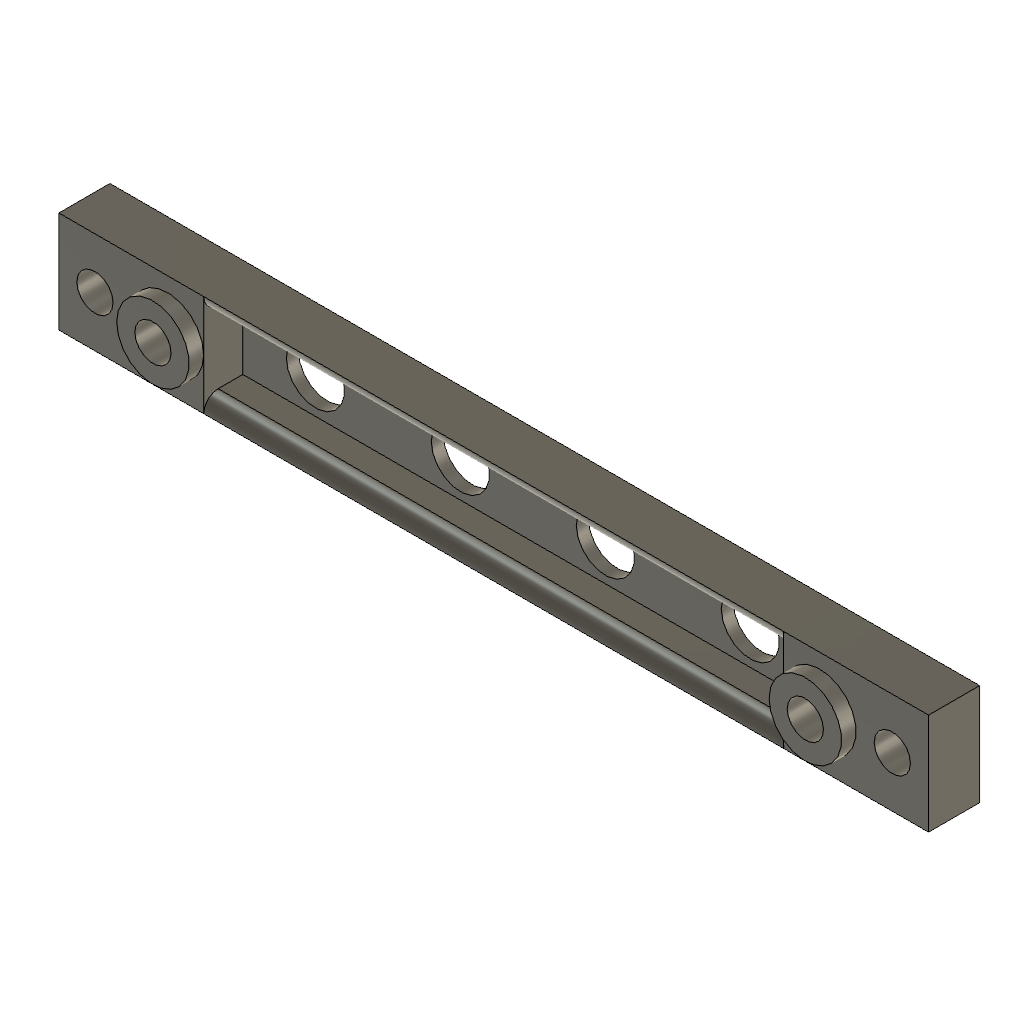
Button Plate (Autodesk Fusion 360 design; units mm, degrees)
Autodesk Fusion 360 part; units mm, degrees
note: some values were not read from the file. Set by a fixed rule: which sketch regions a step uses.
sketch "Sketch1" plane through (0, 0, 0) normal (0, 1, 0) x (1, 0, 0)
  line L0 (0, 0) -> (60, 0)
  line L1 (60, 0) -> (60, -7)
  line L2 (60, -7) -> (0, -7)
  line L3 (0, -7) -> (0, 0)
  line L4 (0, -7) -> (2.5, -7)
  line L5 (2.5, -7) -> (2.5, -3.5)
  line L6 (2.5, -3.5) -> (0, -3.5)
  line L7 (0, -3.5) -> (0, -7)
  line L8 (60, -7) -> (57.5, -7)
  line L9 (57.5, -7) -> (57.5, -3.5)
  line L10 (57.5, -3.5) -> (60, -3.5)
  line L11 (60, -3.5) -> (60, -7)
  circle A0 centre (2.5, -3.5) radius 1.25
  circle A1 centre (57.5, -3.5) radius 1.25
  line L12 (0, -7) -> (30, -7)
  line L13 (0, -7) -> (18, -7)
  line L14 (60, -7) -> (42, -7)
  line L15 (2.5, -3.5) -> (7.5, -3.5)
  line L16 (57.5, -3.5) -> (52.5, -3.5)
  circle A2 centre (7.5, -3.5) radius 1.25
  circle A3 centre (52.5, -3.5) radius 1.25
  circle A4 centre (52.5, -3.5) radius 2.5
  circle A5 centre (7.5, -3.5) radius 2.5
  line L17 (7.5, -3.5) -> (15, -3.5)
  line L18 (52.5, -3.5) -> (45, -3.5)
  line L19 (15, -3.5) -> (25, -3.5)
  line L20 (25, -3.5) -> (35, -3.5)
  line L21 (35, -3.5) -> (45, -3.5)
  circle A6 centre (15, -3.5) radius 2
  circle A7 centre (25, -3.5) radius 2
  circle A8 centre (35, -3.5) radius 2
  circle A9 centre (45, -3.5) radius 2
  dimension "d1" = 60
  dimension "d2" = 7
  dimension "d3" = 2.5
  dimension "d4" = 3.5
  dimension "d5" = 2.5
  dimension "d6" = 3.5
  dimension "d7" = 2.5
  dimension "d8" = 2.5
  dimension "d79" = 5
  dimension "d80" = 5
  dimension "d81" = 2.5
  dimension "d82" = 2.5
  dimension "d83" = 5
  dimension "d84" = 5
  dimension "d85" = 7.5
  dimension "d86" = 7.5
  dimension "d87" = 10
  dimension "d88" = 10
  dimension "d89" = 10
  dimension "d90" = 4
  dimension "d91" = 4
  dimension "d92" = 4
  dimension "d93" = 4
  constraint horizontal L0
  constraint vertical L1
  constraint horizontal L2
  constraint vertical L3
  constraint coincident L0.start L3.end
  constraint horizontal L4
  constraint vertical L5
  constraint horizontal L6
  constraint vertical L7
  constraint horizontal L8
  constraint vertical L9
  constraint horizontal L10
  constraint vertical L11
  constraint coincident L5.end L6.start
  constraint coincident L9.end L10.start
  constraint perpendicular L7 L12
  constraint perpendicular L5 L13
  constraint perpendicular L11 L14
  constraint perpendicular L5 L15
  constraint perpendicular L9 L16
  constraint coincident L15.end A2.centre
  constraint coincident L16.end A3.centre
  constraint concentric A3 A4
  constraint concentric A2 A5
  constraint parallel L15 L17
  constraint parallel L16 L18
  constraint parallel L17 L19
  constraint parallel L19 L20
  constraint parallel L20 L21
  constraint coincident L17.end L19.start
  constraint coincident L19.end L20.start
  constraint coincident L20.end L21.start
  constraint coincident L18.end L21.end
  measures "d1" distance of L0.start L0.end
  measures "d2" distance of L0.start L2.end
  measures "d3" distance of L2.end L4.end
  measures "d4" distance of L2.end L6.end
  measures "d5" distance of L1.end L8.end
  measures "d6" distance of L1.end L10.end
  measures "d7" diameter of A0
  measures "d8" diameter of A1
  measures "d79" distance of L5.end L15.end
  measures "d80" distance of L9.end L16.end
  measures "d81" diameter of A2
  measures "d82" diameter of A3
  measures "d83" diameter of A4
  measures "d84" diameter of A5
  measures "d85" distance of L15.end L17.end
  measures "d86" distance of L16.end L18.end
  measures "d87" distance of L17.end L19.end
  measures "d88" distance of L19.end L20.end
  measures "d89" distance of L20.end L18.end
  measures "d90" diameter of A6
  measures "d91" diameter of A7
  measures "d92" diameter of A8
  measures "d93" diameter of A9
extrude "Extrude1" add sketch "Sketch1" along normal blind 3.532 contours L0 L1 L3 L6 L10 A0 A1 L15 L16 A4 A5 L17 L18 L19 L20 L21 A6 A7 A8 A9 | L2 L3 L4 L5 L6 L7 A0 L12 L13 | L1 L2 L8 L9 L10 L11 A1 L14 | L6 A0 L15 | L5 L6 A0 | L9 L10 A1 | L10 A1 L16 | L2 L5 L9 A0 A1 L12 L13 L14 L15 L16 A4 A5 L17 L18 L19 L20 L21 A6 A7 A8 A9 | L5 A0 L15 | L9 A1 L16 | L15 A2 A5 L17 | L15 A2 A5 L17 | L16 A3 A4 L18 | L16 A3 A4 L18 | L15 A2 L17 | L15 A2 L17 | L16 A3 L18 | L16 A3 L18
extrude "Extrude3" cut sketch "Sketch1" along normal blind 2 contours L6 A0 L15 | L5 L6 A0 | L9 L10 A1 | L10 A1 L16 | L5 A0 L15 | L9 A1 L16
extrude "Extrude4" add sketch "Sketch1" against normal blind 1 contours L15 A2 A5 L17 | L15 A2 A5 L17 | L16 A3 A4 L18 | L16 A3 A4 L18
extrude "Extrude12" cut 2 faces at (52.6522, 0, 3.8879) (7.2402, 0, 3.8258) along direction (0, 1, 0) blind 2
sketch "Sketch5" plane through (0, 0, 0) normal (0, -1, 0) x (1, 0, 0)
  circle A0 centre (7.5, 3.5) radius 2.5
  circle A1 centre (2.5, 3.5) radius 1.25
  circle A2 centre (57.5, 3.5) radius 1.25
  circle A3 centre (15, 3.5) radius 2
  circle A4 centre (45, 3.5) radius 2
  circle A5 centre (25, 3.5) radius 2
  circle A6 centre (35, 3.5) radius 2
  line L0 (0, 7) -> (0, 0)
  line L1 (0, 0) -> (60, 0)
  line L2 (60, 0) -> (60, 7)
  line L3 (60, 7) -> (0, 7)
  circle A7 centre (52.5, 3.5) radius 2.5
  line L4 (10, 3.5) -> (10, 7)
  line L5 (10, 7) -> (50, 7)
  line L6 (50, 7) -> (50, 0)
  line L7 (50, 0) -> (10, 0)
  line L8 (10, 0) -> (10, 7)
  line L9 (10, 7) -> (50, 7)
  line L10 (50, 7) -> (50, 6)
  line L11 (50, 6) -> (10, 6)
  line L12 (10, 6) -> (10, 7)
  line L13 (10, 0) -> (50, 0)
  line L14 (50, 0) -> (50, 1)
  line L15 (50, 1) -> (10, 1)
  line L16 (10, 1) -> (10, 0)
  dimension "d94" = 1
  constraint coincident A0 L4.start
  constraint coincident L3 L4.end
  constraint tangent A0 L4
  constraint perpendicular L3 L4
  constraint horizontal L5
  constraint vertical L6
  constraint horizontal L7
  constraint vertical L8
  constraint coincident L1 L6.end
  constraint horizontal L9
  constraint vertical L10
  constraint horizontal L11
  constraint vertical L12
  constraint horizontal L13
  constraint vertical L14
  constraint horizontal L15
  constraint vertical L16
  constraint coincident L6 L14.end
  measures "d94" distance of L4.end L11.end
extrude "Extrude11" cut sketch "Sketch5" against normal blind 2.7 contours L4 L6 L8 L11 L15
fillet "Fillet4" radius 1 2 edges at (30, 0, 6) (30, 0, 1)
